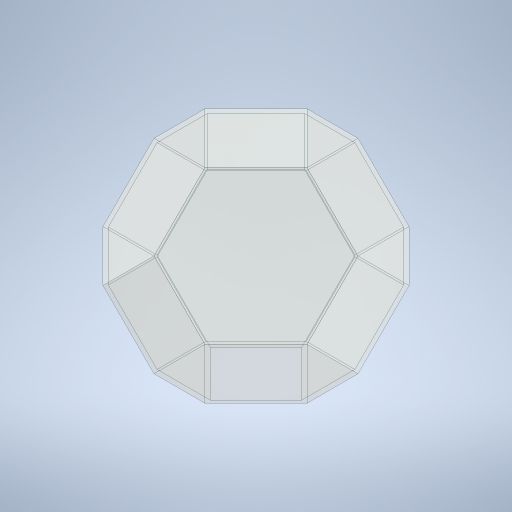
# Autodesk Inventor part: Dome
Saved by Autodesk Inventor 2024 (Build 280153000, 153)
## iProperties
Created: 2023-06-28
Part Number: Dome
Material: Glass
Document SubType Name: Modeling
Designer: jrese
Density: 2.18 g/cm^3
Appearance: Clear
Author: jrese
Autodesk Inventor part; units mm, degrees
ref_plane "YZ Plane" through (0, 0, 0) normal (1, 0, 0) x (0, 1, 0)
ref_plane "XZ Plane" through (0, 0, 0) normal (0, 1, 0) x (-1, 0, 0)
sketch "Sketch26" plane through (0, 0, 0) normal (0, 0, 1) x (1, 0, 0)
  line L0 (82.5476, 0) -> (0, 82.5476)
  line L1 (0, 82.5476) -> (-82.5476, 0)
  line L2 (-82.5476, 0) -> (0, -82.5476)
  line L3 (0, -82.5476) -> (82.5476, 0)
  line L4 (-58.37, -58.37) -> (58.37, 58.37) construction
  line L5 (58.37, -58.37) -> (-58.37, 58.37) construction
  point P0 (0, 0)
  dimension "d97" = 116.74
  dimension "d98" = 165.0953
  constraints: 12 end point, 2 midpoint, 2 parallel, 1 perpendicular
  measures "d97" distance of L0.end L1.end
  measures "d98" distance of L0.start L1.end
extrude "Extrusion9" add sketch "Sketch26" along normal mid plane 330.1906
pattern_circular "Circular Pattern14" count 4 over 360 about axis through (-10, 0, 0) along (1, 0, 0) of "Extrusion9"
pattern_circular "Circular Pattern15" count 4 over 360 about axis through (0, -10, 0) along (0, 1, 0) of "Extrusion9"
ref_plane "Work Plane9" through (82.5476, 165.0953, 0) normal (0.5773503, 0.5773503, 0.5773503) x (0.7071068, 0, -0.7071068)
sketch "Sketch27" plane through (82.5476, 165.0953, 0) normal (0.5773503, 0.5773503, 0.5773503) x (0.7071068, 0, -0.7071068)
  line L0 (-116.74, -67.3999) -> (-116.74, 0) projected
  line L1 (-116.74, 0) -> (0, 0)
  line L2 (0, 0) -> (58.37, -101.0998)
  line L3 (58.37, -101.0998) -> (0, -202.1996)
  line L4 (0, -202.1996) -> (-116.74, -202.1996)
  line L5 (-116.74, -202.1996) -> (-175.11, -101.0998)
  line L6 (-175.11, -101.0998) -> (-116.74, 0)
  point P0 (-58.37, -101.0998)
  point P1 (-58.37, -101.0998)
  constraints: 12 end point, 1 coincident, 13 other
extrude "Extrusion10" add sketch "Sketch27" against normal up to surface (285.9534 mm away)
pattern_circular "Circular Pattern16" count 4 over 360 about axis through (-10, 0, 0) along (1, 0, 0) of "Extrusion10"
shell "Shell2" thickness 5 removed faces 1 at (0, -165.0953, -27.5159)
equation "\"d99\" = 2 * d98"
equation "\"d107\" = 2 * d98"
body "Solid7"
